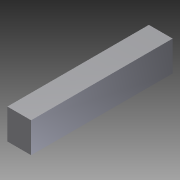
# Autodesk Inventor part: key for pneumatic wheel + motor
Saved by Autodesk Inventor 2011 SP1 (Build 150282100, 282)
## iProperties
Created: 2013-01-18
Part Number: key for pneumatic wheel + motor
Document SubType Name: Modeling
Designer: wes
Density: 1 g/cm^3
Author: wes
Autodesk Inventor part; units mm, degrees
ref_plane "YZ Plane" through (0, 0, 0) normal (1, 0, 0) x (0, 1, 0)
ref_plane "XZ Plane" through (0, 0, 0) normal (0, 1, 0) x (-1, 0, 0)
ref_plane "XY Plane" through (0, 0, 0) normal (0, 0, 1) x (1, 0, 0)
sketch "Sketch1" plane through (0, 0, 0) normal (0, 0, 1) x (1, 0, 0)
  line L0 (-15.5357, -3.6826) -> (-12.3353, -3.6826)
  line L1 (-12.3353, -3.6826) -> (-12.3353, 0.3814)
  line L2 (-12.3353, 0.3814) -> (-15.5357, 0.3814)
  line L3 (-15.5357, 0.3814) -> (-15.5357, -3.6826)
  point P0 (0, 0)
  dimension "d0" = 4.064
  dimension "d1" = 3.2004
  constraints: 8 end point, 2 parallel, 1 horizontal, 1 perpendicular
  measures "d0" distance of L0.end L1.end
  measures "d1" distance of L0.start L0.end
extrude "Extrusion1" add sketch "Sketch1" along normal blind 19.05
body "Solid1"
